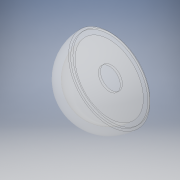
# Autodesk Inventor part: kaca
Saved by Autodesk Inventor 2019.5 (Build 235369000, 369)
## iProperties
Created: 2022-10-11
Part Number: kaca
Material: Polycarbonate, Clear
Document SubType Name: Modeling
Designer: ASUS
Density: 1.2 g/cm^3
Appearance: Polycarbonate - Clear
Author: ASUS
Autodesk Inventor part; units mm, degrees
ref_plane "YZ Plane" through (0, 0, 0) normal (1, 0, 0) x (0, 1, 0)
ref_plane "XZ Plane" through (0, 0, 0) normal (0, 1, 0) x (-1, 0, 0)
ref_plane "XY Plane" through (0, 0, 0) normal (0, 0, 1) x (1, 0, 0)
sketch "Sketch1" plane through (0, 0, 0) normal (0, 0, 1) x (1, 0, 0)
  arc A0 (20.6974, 35.3693) -> (20.6974, 72.3693) centre (20.6974, 53.8693) ccw
  line L0 (20.6974, 72.3693) -> (20.6974, 35.3693)
  circle A1 centre (20.6974, 53.8693) radius 17.5
  point P0 (0, 0)
  dimension "d0" = 37
  dimension "d2" = 35
  constraints: 2 centre point, 2 end point, 2 point on circle, 1 coincident
  measures "d0" diameter of A0
  measures "d2" diameter of A1
revolve "Revolution1" add sketch "Sketch1" angle 180 about axis through (20.6974, 72.3693, 0) along (0, -1, 0) picked at (29.7821, 55.9689) contours L0 A1 A0 | L0 A1
shell "Shell2" thickness 3 removed faces 1 at (14.9315, 56.056, 0)
extrude "Extrusion3" add sketch "Sketch1" against normal blind 1 contours A1 L0 | L0 A1
hole "Hole3" at (20.6974, 53.8693, 0) direction (0, 0, -1) diameter 10 depth 1
body "Solid1"
